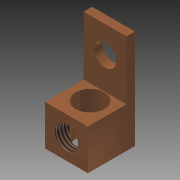
# Autodesk Inventor part: Terminal Battery
Saved by Autodesk Inventor 2013 (Build 170138000, 138)
## iProperties
Shininess: 64.0
Angle Display Precision: 2
Document Length Units: 11269
Document Angle Units: 11279
Document Time Units: 11290
Document Mass Units: 11283
Document Length Units Precision: 3
Document Angle Units Precision: 2
Created: 2003-03-14
Part Number: Terminal Battery
Material: Copper
Document SubType Name: Modeling
Designer: t8558es
Vendor: FCI Burndy
Density: 1 g/cm^3
Density: 0.0
Volumn: 0.0
Area: 0.0
PropertySet Name: Model Information
Control State: 0
Master: False
Checked Out: False
Author: t8558es
Autodesk Inventor part; units mm, degrees
ref_plane "YZ Plane" through (0, 0, 0) normal (1, 0, 0) x (0, 1, 0)
ref_plane "XZ Plane" through (0, 0, 0) normal (0, 1, 0) x (-1, 0, 0)
ref_plane "XY Plane" through (0, 0, 0) normal (0, 0, 1) x (1, 0, 0)
sketch "Sketch1" plane through (0, 0, 0) normal (0, 0, 1) x (1, 0, 0)
  line L0 (-11.9586, 8.8362) -> (0.7914, 8.8362)
  line L1 (0.7914, 8.8362) -> (0.7914, -5.1638)
  line L2 (0.7914, -5.1638) -> (-11.9586, -5.1638)
  line L3 (-11.9586, -5.1638) -> (-11.9586, 8.8362)
  circle A0 centre (-5.5836, 1.8362) radius 4.2944
  dimension "d0" = 12.75
  dimension "d1" = 14
  dimension "d2" = 6.375
  dimension "d3" = 7
  constraints: 8 end point, 2 parallel, 1 centre point, 1 horizontal, 1 perpendicular
  measures "d0" distance of L0.start L0.end
  measures "d1" distance of L2.end L0.start
  measures "d2" distance from line of L1 A0.centre
  measures "d3" distance from line of L0 A0.centre
extrude "Extrusion1" add sketch "Sketch1" along normal blind 12
sketch "Sketch2" plane through (0, 0, 12) normal (0, 0, 1) x (1, 0, 0)
  line L0 (0.7914, 8.8362) -> (0.7914, -5.1638) projected
  line L1 (-11.9586, 8.8362) -> (0.7914, 8.8362) projected
  line L2 (-11.9586, -5.1638) -> (-11.9586, 8.8362) projected
  line L3 (-11.9586, 6.3362) -> (0.7914, 6.3362)
  dimension "d7" = 2.5
  constraints: 2 end point, 2 point on line, 1 parallel
  measures "d7" distance between parallel lines of L3 L1
extrude "Extrusion2" add sketch "Sketch2" along normal blind 17.5
sketch "Sketch3" plane through (-11.9586, 6.3362, 12) normal (0, -1, 0) x (1, 0, 0)
  line L0 (12.75, 17.5) -> (0, 17.5) projected
  line L1 (0, 0) -> (0, 17.5) projected
  point P0 (6.375, 9.5)
  dimension "d10" = 8
  dimension "d11" = 6.375
  measures "d10" distance from line of L0 point (6.375, 9.5)
  measures "d11" distance from line of L1 point (6.375, 9.5)
hole "Hole1" at (-5.5836, 6.3362, 21.5) direction (0, 1, 0) diameter 6.5 end through all
sketch "Sketch4" plane through (-11.9586, -5.1638, 0) normal (0, -1, 0) x (1, 0, 0)
  line L0 (12.75, 12) -> (0, 12) projected
  line L1 (0, 0) -> (0, 12) projected
  point P0 (6.375, 6)
  dimension "d19" = 6.375
  dimension "d20" = 6
  measures "d19" distance from line of point (6.375, 6) L1
  measures "d20" distance from line of point (6.375, 6) L0
hole "Hole2" at (-5.5836, -5.1638, 6) direction (0, 1, 0) diameter 6.917 depth 7 tip angle 118 thread size "M8x1" class "6H" standard "ANSI Metric M Profile"
equation "\"d2\" = 0.5 * d0"
equation "\"d3\" = 0.5 * d1"
equation "\"d11\" = 0.5 * d0"
equation "\"d19\" = 0.5 * d0"
body "Solid1"
